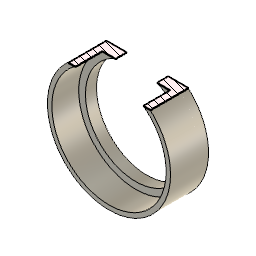
Mount (Autodesk Fusion 360 design; units mm, degrees)
Autodesk Fusion 360 part; units mm, degrees
note: some values were not read from the file. Set by a fixed rule: which sketch regions a step uses.
sketch "Sketch1" plane through (0, 0, 0) normal (0, 1, 0) x (1, 0, 0)
  circle A0 centre (-16.131, -18.3661) radius 25.5
  circle A1 centre (108.869, -18.3661) radius 25.5
  dimension "d1" = 51
  dimension "d2" = 125
  dimension "d3" = 51
  measures "d1" diameter of A0
  measures "d2" distance of A0.centre A1.centre
  measures "d3" diameter of A1
extrude "Extrude1" add sketch "Sketch1" along normal blind 15 makes body 1 at (9.2422, 10, 20.905) makes body 2 at (134.2422, 10, 20.905)
extrude "Extrude2" add 1 faces at (116.5272, 15, 14.6781) along direction (0, 1, 0) blind 4 on bodies 2 bodies 2
sketch "Sketch2" plane through (0, 0, 0) normal (0, 1, 0) x (1, 0, 0)
sketch "Sketch3" plane through (0, 0, 0) normal (0, -1, 0) x (1, 0, 0)
  circle A0 centre (-16.131, 18.3661) radius 25.5
  line L0 (-16.131, 53.8661) -> (108.869, 53.8661)
  line L1 (108.869, -17.1339) -> (-16.131, -17.1339)
  line L2 (-16.131, 53.8661) -> (-66.131, 53.8661)
  line L3 (-66.131, 53.8661) -> (-66.131, -17.1339)
  line L4 (-66.131, -17.1339) -> (-16.131, -17.1339)
  line L5 (108.869, 53.8661) -> (158.869, 53.8661)
  line L6 (158.869, 53.8661) -> (158.869, -17.1339)
  line L7 (158.869, -17.1339) -> (108.869, -17.1339)
  circle A1 centre (108.869, 18.3661) radius 25.25
  circle A2 centre (-16.131, 18.3661) radius 25.25
  dimension "d10" = 125
  dimension "d11" = 71
  dimension "d12" = 50
  dimension "d13" = 50
  dimension "d14" = 50.5
  dimension "d15" = 125
  dimension "d16" = 50.5
  constraint horizontal L0
  constraint horizontal L1
  constraint horizontal L2
  constraint vertical L3
  constraint horizontal L4
  constraint horizontal L5
  constraint vertical L6
  constraint horizontal L7
  measures "d10" distance of L0.start L0.end
  measures "d11" distance of L0.start L1.end
  measures "d12" distance of L0.start L2.end
  measures "d13" distance of L0.end L5.end
  measures "d14" diameter of A1
  measures "d15" distance of A1.centre A0.centre
  measures "d16" diameter of A2
extrude "Extrude3" add sketch "Sketch3" against normal blind 4 separate body contours L0 L1 L2 L3 L4 L5 L6 L7 makes body 3
sketch "Sketch4" plane through (0, 4, 0) normal (0, 1, 0) x (-1, 0, 0)
  circle A0 centre (16.131, 18.3661) radius 25.5
  circle A1 centre (-108.869, 18.3661) radius 25.25
  line L0 (66.131, 53.8661) -> (-158.869, 53.8661)
  line L1 (-158.869, 53.8661) -> (-158.869, -17.1339)
  line L2 (-158.869, -17.1339) -> (66.131, -17.1339)
  line L3 (66.131, -17.1339) -> (66.131, 53.8661)
  line L4 (-158.869, -17.1339) -> (66.131, -17.1339)
  line L5 (66.131, -17.1339) -> (66.131, -12.1339)
  line L6 (66.131, -12.1339) -> (-158.869, -12.1339)
  line L7 (-158.869, -12.1339) -> (-158.869, -17.1339)
  dimension "d19" = 5
  constraint horizontal L4
  constraint vertical L5
  constraint horizontal L6
  constraint vertical L7
  constraint coincident L1.end L2.start
  measures "d19" distance of L1.end L6.end
extrude "Extrude4" add sketch "Sketch4" along normal blind 35 contours L1 L2 L3 L4 L5 L6 L7 bodies 3
sketch "Sketch5" plane through (-66.131, 0, 0) normal (-1, 0, 0) x (0, -1, 0)
  line L0 (0, -17.1339) -> (0, 53.8661)
  line L1 (0, 53.8661) -> (-4, 53.8661)
  line L2 (-4, 53.8661) -> (-4, -12.1339)
  line L3 (-4, -12.1339) -> (-39, -12.1339)
  line L4 (-39, -12.1339) -> (-39, -17.1339)
  line L5 (-39, -17.1339) -> (0, -17.1339)
  line L6 (0, -17.1339) -> (-39, -17.1339)
  line L7 (-39, -17.1339) -> (-39, 53.8661)
  line L8 (-39, 53.8661) -> (0, 53.8661)
  line L9 (0, 53.8661) -> (0, -17.1339)
  dimension "d22" = 39
  constraint horizontal L6
  constraint vertical L7
  constraint horizontal L8
  constraint vertical L9
  constraint coincident L0.start L5.end
  measures "d22" distance of L0.start L4.end
extrude "Extrude5" add sketch "Sketch5" against normal blind 5 contours L2 L3 L7 L8 bodies 3
sketch "Sketch6" plane through (158.869, 0, 0) normal (1, 0, 0) x (0, 1, 0)
  line L0 (0, 53.8661) -> (0, -17.1339)
  line L1 (0, -17.1339) -> (39, -17.1339)
  line L2 (39, -17.1339) -> (39, -12.1339)
  line L3 (39, -12.1339) -> (4, -12.1339)
  line L4 (4, -12.1339) -> (4, 53.8661)
  line L5 (4, 53.8661) -> (0, 53.8661)
  line L6 (0, -17.1339) -> (39, -17.1339)
  line L7 (39, -17.1339) -> (39, 53.8661)
  line L8 (39, 53.8661) -> (0, 53.8661)
  line L9 (0, 53.8661) -> (0, -17.1339)
  dimension "d25" = 39
  constraint horizontal L6
  constraint vertical L7
  constraint horizontal L8
  constraint vertical L9
  constraint coincident L0.end L1.start
  measures "d25" distance of L0.end L1.end
extrude "Extrude6" add sketch "Sketch6" against normal blind 5 contours L3 L4 L7 L8 bodies 3
fillet "Fillet1" radius 2 6 edges at (-66.131, 19.5, 53.8661) (46.369, 0, 53.8661) (-66.131, 0, 18.3661) (158.869, 19.5, 53.8661) (158.869, 0, 18.3661) (46.369, 0, -17.1339) on bodies 3
fillet "Fillet2" radius 1 2 edges at (-39.9054, 0, 27.5873) (85.3277, 0, 27.4969) on bodies 3
sketch "Sketch7" plane through (0, 4, 0) normal (0, 1, 0) x (-1, 0, 0)
  circle A0 centre (-108.869, 18.3661) radius 25.25
  circle A1 centre (16.131, 18.3661) radius 25.5
  line L0 (-153.869, 53.8661) -> (-153.869, -12.1339)
  line L1 (-153.869, -12.1339) -> (61.131, -12.1339)
  line L2 (61.131, -12.1339) -> (61.131, 53.8661)
  line L3 (61.131, 53.8661) -> (-153.869, 53.8661)
  line L4 (-153.869, 53.8661) -> (61.131, 53.8661)
  line L5 (61.131, 53.8661) -> (61.131, 49.8661)
  line L6 (61.131, 49.8661) -> (-153.869, 49.8661)
  line L7 (-153.869, 49.8661) -> (-153.869, 53.8661)
  dimension "d32" = 215
  dimension "d33" = 4
  constraint horizontal L4
  constraint vertical L5
  constraint horizontal L6
  constraint vertical L7
  constraint coincident L0.start L3.end
  measures "d32" distance of L0.start L2.end
  measures "d33" distance of L0.start L6.end
extrude "Extrude7" add sketch "Sketch7" along normal blind 35 contours L0 L2 L3 L4 L5 L6 L7 bodies 3
sketch "Sketch8" plane through (0, 0, 53.8661) normal (0, 0, 1) x (-1, 0, 0)
  line L0 (-156.869, -2) -> (-156.869, -39)
  line L1 (-156.869, -39) -> (64.131, -39)
  line L2 (64.131, -39) -> (64.131, -2)
  line L3 (64.131, -2) -> (-156.869, -2)
  circle A0 centre (-126.369, -20.5) radius 2.5
  circle A1 centre (33.631, -20.5) radius 2.5
  dimension "d37" = 5
  dimension "d38" = 5
  measures "d37" diameter of A0
  measures "d38" diameter of A1
extrude "Extrude8" cut sketch "Sketch8" against normal blind 200 contours A0 | A1 bodies 3
sketch "Sketch9" plane through (0, 4, 0) normal (0, 1, 0) x (-1, 0, 0)
  line L0 (61.131, 49.8661) -> (-153.869, 49.8661)
  line L1 (-153.869, 49.8661) -> (-153.869, -12.1339)
  line L2 (-153.869, -12.1339) -> (61.131, -12.1339)
  line L3 (61.131, -12.1339) -> (61.131, 49.8661)
  circle A0 centre (16.131, 18.3661) radius 25.5
  circle A1 centre (-108.869, 18.3661) radius 25.25
  circle A2 centre (-108.869, 18.3661) radius 27.5
  circle A3 centre (-108.869, 18.3661) radius 25.25
  circle A4 centre (16.131, 18.3661) radius 27.5
  circle A5 centre (16.131, 18.3661) radius 25.5
  dimension "d41" = 55
  dimension "d42" = 55
  constraint concentric A1 A2
  constraint concentric A2 A3
  constraint concentric A0 A4
  constraint concentric A4 A5
  measures "d41" diameter of A2
  measures "d42" diameter of A4
extrude "Extrude9" add sketch "Sketch9" along normal blind 15 separate body contours A2 | A4 makes body 4 at (81.5056, 14, 15.6279) makes body 5 at (-43.4944, 14, 15.6279)
sketch "Sketch10" plane through (0, 19, 0) normal (0, 1, 0) x (-1, 0, 0)
  circle A0 centre (16.131, 18.3661) radius 25.5
  circle A1 centre (16.131, 18.3661) radius 27.5
  circle A2 centre (16.131, 18.3661) radius 22.5
  circle A3 centre (16.131, 18.3661) radius 27.5
  dimension "d45" = 45
  dimension "d46" = 55
  constraint concentric A0 A2
  constraint concentric A2 A3
  measures "d45" diameter of A2
  measures "d46" diameter of A3
extrude "Extrude10" add sketch "Sketch10" along normal blind 5 contours A0 | A1 A3 bodies 5
sketch "Sketch11" plane through (0, 19, 0) normal (0, 1, 0) x (-1, 0, 0)
  circle A0 centre (-108.869, 18.3661) radius 25.25
  circle A1 centre (-108.869, 18.3661) radius 27.5
  circle A2 centre (-108.869, 18.3661) radius 22.5
  circle A3 centre (-108.869, 18.3661) radius 27.5
  circle A4 centre (-108.869, 18.3661) radius 27.5
  circle A5 centre (-108.869, 18.3661) radius 27.5
  dimension "d49" = 45
  dimension "d50" = 55
  constraint concentric A0 A2
  constraint concentric A2 A3
  constraint concentric A3 A4
  constraint concentric A2 A5
  measures "d49" diameter of A2
  measures "d50" diameter of A5
extrude "Extrude11" add sketch "Sketch11" along normal blind 5 contours A0 | A1 A3 A4 A5 bodies 4
sketch "Sketch12" plane through (0, 39, 0) normal (0, 1, 0) x (-1, 0, 0)
  line L0 (61.131, 49.8661) -> (61.131, -12.1339)
  line L1 (61.131, -12.1339) -> (-153.869, -12.1339)
  line L2 (-153.869, -12.1339) -> (-153.869, 49.8661)
  line L3 (-153.869, 49.8661) -> (61.131, 49.8661)
  line L4 (64.131, 53.8661) -> (-156.869, 53.8661)
  arc A0 (-156.869, 53.8661) -> (-158.869, 51.8661) centre (-156.869, 51.8661) ccw
  line L5 (-158.869, 51.8661) -> (-158.869, -17.1339)
  line L6 (-158.869, -17.1339) -> (66.131, -17.1339)
  line L7 (66.131, -17.1339) -> (66.131, 51.8661)
  arc A1 (66.131, 51.8661) -> (64.131, 53.8661) centre (64.131, 51.8661) ccw
  line L8 (-158.869, 53.8661) -> (66.131, 53.8661)
  line L9 (66.131, 53.8661) -> (66.131, -17.1339)
  line L10 (66.131, -17.1339) -> (-158.869, -17.1339)
  line L11 (-158.869, -17.1339) -> (-158.869, 53.8661)
  constraint horizontal L8
  constraint vertical L9
  constraint horizontal L10
  constraint vertical L11
  constraint coincident L6.end L7.start
extrude "Extrude12" add sketch "Sketch12" along normal mid plane 10 separate body contours L0 L1 L2 L3 | L4 A0 L5 L6 L7 A1 L8 L9 L10 L11 makes body 6
extrude "Extrude13" cut 1 faces at (10.5356, 39, -15.4673) along direction (0, -1, 0) up to surface (5 mm away) on bodies 3 bodies 6
sketch "Sketch13" plane through (0, 34, 0) normal (0, -1, 0) x (1, 0, 0)
  line L0 (153.869, 49.8661) -> (-61.131, 49.8661)
  line L1 (-61.131, 49.8661) -> (-61.131, -12.1339)
  line L2 (-61.131, -12.1339) -> (153.869, -12.1339)
  line L3 (153.869, -12.1339) -> (153.869, 49.8661)
  line L4 (51.369, -12.1339) -> (51.369, -17.1339)
  line L5 (51.369, -17.1339) -> (41.369, -17.1339)
  line L6 (41.369, -17.1339) -> (41.369, -12.1339)
  arc A0 (51.369, -12.1339) -> (41.369, -12.1339) centre (46.369, -12.1339) ccw
  dimension "d57" = 10
  dimension "d58" = 10
  dimension "d59" = 5
  constraint midpoint L2 A0.centre
  constraint vertical L4
  constraint horizontal L5
  constraint vertical L6
  constraint coincident L2 L6.end
  measures "d57" diameter of A0
  measures "d58" distance of L6.end L4.start
  measures "d59" distance of L6.end L5.end
extrude "Extrude14" cut sketch "Sketch13" against normal blind 20 contours L2 L4 L5 L6 | L2 A0 bodies 6
extrude "Extrude15" cut 1 faces at (-42.7671, 4, 15.733) along direction (0, 1, 0) blind 3 on bodies 5 bodies 5
move_body "Move1" bodies 5 to x (1, 0, 0) y (0, 1, 0) z (0, 0, 1) at (0, -3, 0)
sketch "Sketch14" plane through (0, 0, 53.8661) normal (0, 0, 1) x (-1, 0, 0)
  circle A0 centre (-126.369, -20.5) radius 2.5
  circle A1 centre (33.631, -20.5) radius 2.5
  line L0 (-156.869, -2) -> (-156.869, -39)
  line L1 (-156.869, -39) -> (64.131, -39)
  line L2 (64.131, -39) -> (64.131, -2)
  line L3 (64.131, -2) -> (-156.869, -2)
  line L4 (-156.869, -20.5) -> (64.131, -20.5)
  circle A2 centre (53.631, -20.5) radius 2.5
  circle A3 centre (-146.369, -20.5) radius 2.5
  dimension "d66" = 5
  dimension "d67" = 5
  constraint midpoint L0 L4.start
  constraint midpoint L2 L4.end
  constraint coincident L4 A2.centre
  constraint coincident L4 A3.centre
  measures "d66" diameter of A2
  measures "d67" diameter of A3
extrude "Extrude16" cut sketch "Sketch14" against normal blind 200 contours L4 A3 | L4 A3 | L4 A2 | L4 A2 bodies 3
hidden bodies 1 2 3 4 6
named bodies: "Red", "Green", "Base", "Mount", "Mount 2"
